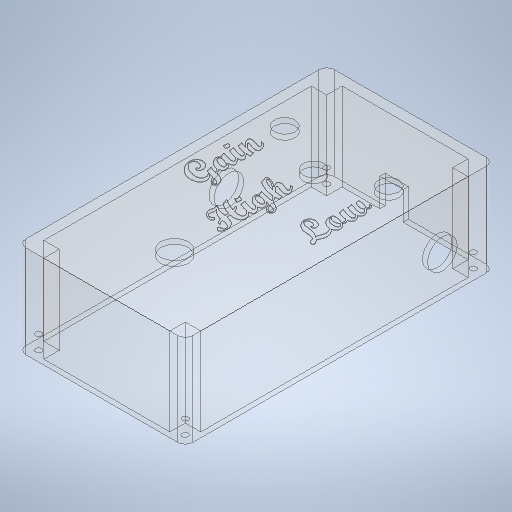
# Autodesk Inventor part: obudowa
Saved by Autodesk Inventor 2025 (Build 290162000, 162)
## iProperties
Created: 2026-04-02
Part Number: obudowa
Material: Tworzywo sztuczne PET
Document SubType Name: Modeling
Designer: zzapa
Density: 1.541 g/cm^3
Appearance: Poliwęglan — przezroczysty
Author: zzapa
Autodesk Inventor part; units mm, degrees
note: some values were not read from the file. Chosen so that the rebuilt part matches the saved one: direction of "JACK 2"; direction of "JACK 1".
ref_plane "YZ Plane" through (0, 0, 0) normal (1, 0, 0) x (0, 1, 0)
ref_plane "XZ Plane" through (0, 0, 0) normal (0, 1, 0) x (-1, 0, 0)
sketch "Szkic1" plane through (0, 0, 0) normal (0, 1, 0) x (-1, 0, 0)
  line L0 (65, -120) -> (0, -120)
  line L1 (0, -120) -> (0, 0)
  line L2 (0, 0) -> (65, 0)
  line L3 (65, 0) -> (65, -120)
  dimension "d0" = 120
  dimension "d1" = 65
  constraints: 8 end point, 2 parallel, 1 coincident, 1 horizontal, 1 perpendicular
  measures "d0" distance of L2.end L0.start
  measures "d1" distance of L0.start L0.end
extrude "Gabaryt" add sketch "Szkic1" along normal blind 36
ref_plane "Konstrukcja wycięcia" through (0, 34, 0) normal (0, 1, 0) x (1, 0, 0)
sketch "Szkic2" plane through (0, 0, 0) normal (0, -1, 0) x (1, 0, 0)
  line L0 (-65, 0) -> (0, 0) projected
  line L1 (-65, -120) -> (-65, 0) projected
  line L2 (0, -120) -> (-65, -120) projected
  line L3 (0, 0) -> (0, -120) projected
  line L4 (-2, -118) -> (-63, -118)
  line L5 (-63, -118) -> (-63, -2)
  line L6 (-63, -2) -> (-2, -2)
  line L7 (-2, -2) -> (-2, -118)
  dimension "d4" = 2
  constraints: 8 end point, 3 other
  measures "d4" distance between parallel lines of L3 L7
extrude "Wydrążenie" cut sketch "Szkic2" against normal up to surface (34 mm away) contours L4 L5 L6 L7
sketch "Szkic6" plane through (0, 0, 0) normal (0, -1, 0) x (1, 0, 0)
  line L0 (-65, 0) -> (0, 0) projected
  line L1 (-8, -8) -> (0, -8)
  line L2 (0, -8) -> (0, 0)
  line L3 (0, 0) -> (-8, 0)
  line L4 (-8, 0) -> (-8, -8)
  line L5 (0, 0) -> (0, -120) projected
  line L6 (0, -120) -> (-65, -120) projected
  line L7 (-65, -120) -> (-65, 0) projected
  line L8 (0, 0) -> (0, -120) projected
  line L9 (0, -60) -> (-65, -60)
  line L10 (-32.5, 0) -> (-32.5, -120)
  line L11 (-57, -8) -> (-65, -8)
  line L12 (-65, -8) -> (-65, 0)
  line L13 (-65, 0) -> (-57, 0)
  line L14 (-57, 0) -> (-57, -8)
  line L15 (-8, -112) -> (0, -112)
  line L16 (0, -112) -> (0, -120)
  line L17 (0, -120) -> (-8, -120)
  line L18 (-8, -120) -> (-8, -112)
  line L19 (-57, -112) -> (-65, -112)
  line L20 (-65, -112) -> (-65, -120)
  line L21 (-65, -120) -> (-57, -120)
  line L22 (-57, -120) -> (-57, -112)
  point P0 (-57, -120)
  point P1 (-65, -112)
  point P2 (-57, 0)
  point P3 (-8, -120)
  point P4 (0, -112)
  point P5 (-8, 0)
  dimension "d16" = 8
  dimension "d17" = 8
  constraints: 36 end point, 9 symmetric about line, 4 midpoint, 2 parallel, 1 horizontal, 1 perpendicular
  measures "d16" distance of L1.start L1.end
  measures "d17" distance of L3.end L1.start
extrude "Materiał na insert" add sketch "Szkic6" against normal up to surface (34 mm away) contours L0 L14 L11 L7 | L0 L2 L1 L4 | L19 L22 L6 L7 | L5 L6 L18 L15
sketch "Szkic7" plane through (0, 0, 0) normal (0, -1, 0) x (1, 0, 0)
  line L0 (0, 0) -> (0, -120) projected
  line L1 (0, -60) -> (-65, -60)
  line L2 (-65, -120) -> (-65, 0) projected
  line L3 (0, -120) -> (-65, -120) projected
  line L4 (-32.5, -120) -> (-32.5, 0)
  line L5 (-65, 0) -> (0, 0) projected
  point P0 (-4, -4)
  point P1 (-61, -4)
  point P2 (-4, -116)
  point P3 (-61, -116)
  dimension "d20" = 4
  dimension "d21" = 4
  constraints: 4 end point, 4 midpoint, 3 symmetric about line
  measures "d20" horizontal distance of L0.start point (-4, -4)
  measures "d21" horizontal distance of point (-4, -4) L0.start
hole "Otwory montażowe" at (-4, 0, -4) at (-61, 0, -4) at (-4, 0, -116) at (-61, 0, -116) direction (0, 1, 0) diameter 2.4 depth 5.5
fillet "Zaokrąglenie1" radius 3 4 edges at (-65, 18, 0) (0, 18, 0) (0, 18, -120) (-65, 18, -120)
sketch "Szkic8" plane through (-65, 0, -117) normal (-1, 0, 0) x (0, 0, 1)
  line L0 (-3, 36) -> (-3, 0) projected
  line L1 (0, 0) -> (114, 0) projected
  line L2 (0, 0) -> (-3, 0) projected
  line L3 (117, 0) -> (117, 36) projected
  point P0 (37, 15)
  dimension "d30" = 15
  dimension "d39" = 80
  measures "d30" distance from line of L1 point (37, 15)
  measures "d39" distance from line of L3 point (37, 15)
hole "JACK 1" at (-65, 15, -80) direction (1, 0, 0) diameter 11.5 depth 2
sketch "Szkic9" plane through (0, 0, -3) normal (1, 0, 0) x (0, 0, -1)
  line L0 (0, 0) -> (114, 0) projected
  line L1 (-3, 36) -> (-3, 0) projected
  point P0 (97, 15)
  dimension "d40" = 15
  dimension "d41" = 100
  measures "d40" distance from line of L0 point (97, 15)
  measures "d41" distance from line of point (97, 15) L1
hole "JACK 2" at (0, 15, -100) direction (-1, 0, 0) diameter 11.5 end up to surface
sketch "Szkic11" plane through (0, 36, 0) normal (0, 1, 0) x (1, 0, 0)
  circle A0 centre (-52.7305, 91.416) radius 4
  circle A1 centre (-32.5, 82.3712) radius 4
  line L0 (-3, 120) -> (-62, 120) projected
  line L1 (-32.5, 120) -> (-32.5, 0)
  line L2 (-62, 0) -> (-3, 0) projected
  circle A2 centre (-12.2695, 91.416) radius 4
  circle A3 centre (-32.5, 28.3603) radius 5.3281
  point P0 (0, 0)
  dimension "d51" = 8
  constraints: 4 centre point, 2 end point, 2 midpoint, 2 point on line, 1 equal radius, 1 symmetric about line, 1 other
  measures "d51" diameter of A0
extrude "Wyciągnięcie proste7" cut sketch "Szkic11" against normal up to surface (2 mm away)
sketch "Szkic12" plane through (-3, 0, -120) normal (0, 0, -1) x (-1, 0, 0)
  line L0 (0, 0) -> (59, 0) projected
  line L1 (30.3172, 11) -> (39.3172, 11)
  line L2 (39.3172, 11) -> (39.3172, 0)
  line L3 (39.3172, 0) -> (30.3172, 0)
  line L4 (30.3172, 0) -> (30.3172, 11)
  point P0 (-3, 0)
  point P1 (30.3172, 0)
  dimension "d54" = 11
  dimension "d55" = 9
  constraints: 8 end point, 2 parallel, 1 horizontal, 1 perpendicular, 1 point on line
  measures "d54" distance of L3.end L1.start
  measures "d55" distance of L1.start L1.end
extrude "Wyciągnięcie proste8" cut sketch "Szkic12" against normal up to surface (2 mm away)
sketch "Szkic13" plane through (0, 36, 0) normal (0, 1, 0) x (1, 0, 0)
  line L0 (-60.0879, 47.3044) -> (-60.0879, 81.416) construction
  line L1 (-60.0879, 81.416) -> (-45.3731, 81.416) construction
  line L2 (-45.3731, 81.416) -> (-45.3731, 47.3044) construction
  line L3 (-45.3731, 47.3044) -> (-60.0879, 47.3044) construction
  line L4 (-41.629, 38.2595) -> (-41.629, 72.3712) construction
  line L5 (-41.629, 72.3712) -> (-23.371, 72.3712) construction
  line L6 (-23.371, 72.3712) -> (-23.371, 38.2595) construction
  line L7 (-23.371, 38.2595) -> (-41.629, 38.2595) construction
  line L8 (-20.0288, 47.3044) -> (-20.0288, 81.416) construction
  line L9 (-20.0288, 81.416) -> (-4.5102, 81.416) construction
  line L10 (-4.5102, 81.416) -> (-4.5102, 47.3044) construction
  line L11 (-4.5102, 47.3044) -> (-20.0288, 47.3044) construction
  circle A0 centre (-52.7305, 91.416) radius 4 projected
  circle A1 centre (-32.5, 82.3712) radius 4 projected
  circle A2 centre (-12.2695, 91.416) radius 4 projected
  line L12 (-52.7305, 91.416) -> (-52.7305, 81.416)
  line L13 (-32.5, 82.3712) -> (-32.5, 72.3712)
  line L14 (-12.2695, 91.416) -> (-12.2695, 81.416)
  spline S0 degree 2 poles (-51.1094, 64.0031) (-50.5705, 63.5388) (-49.8905, 62.2121) knots 0 0 0 1 1 1
  spline S1 degree 2 poles (-49.8905, 62.2121) (-48.058, 61.9384) (-46.0514, 60.0479) (-46.0514, 58.8704) knots 0 0 0 1 2 2 2
  spline S2 degree 2 poles (-46.0514, 58.8704) (-46.0514, 58.3066) (-46.5738, 57.6681) (-47.0381, 57.6681) knots 0 0 0 1 2 2 2
  spline S3 degree 2 poles (-47.0381, 57.6681) (-48.3234, 57.6681) (-49.5257, 60.164) knots 0 0 0 1 1 1
  spline S4 degree 2 poles (-49.5257, 60.164) (-50.4544, 60.421) (-51.1924, 60.6698) knots 0 0 0 1 1 1
  spline S5 degree 2 poles (-51.1924, 60.6698) (-50.5705, 60.2303) (-49.6086, 58.5802) (-49.6086, 57.8671) knots 0 0 0 1 2 2 2
  spline S6 degree 2 poles (-49.6086, 57.8671) (-49.6086, 56.7063) (-51.6152, 55.1723) (-53.1492, 55.1723) knots 0 0 0 1 2 2 2
  spline S7 degree 2 poles (-53.1492, 55.1723) (-54.7661, 55.1723) (-57.6683, 56.9053) (-59.4096, 59.7328) (-59.4096, 61.0512) knots 0 0 0 1 2 3 3 3
  spline S8 degree 2 poles (-59.4096, 61.0512) (-59.4096, 62.2369) (-58.058, 63.7212) (-56.9801, 63.7212) knots 0 0 0 1 2 2 2
  spline S9 degree 2 poles (-56.9801, 63.7212) (-55.8275, 63.7212) (-54.0613, 62.0545) (-54.0613, 60.9766) knots 0 0 0 1 2 2 2
  spline S10 degree 2 poles (-54.0613, 60.9766) (-54.0613, 60.3381) (-54.6832, 59.5089) (-55.131, 59.5089) knots 0 0 0 1 2 2 2
  spline S11 degree 2 poles (-55.131, 59.5089) (-55.4129, 59.5089) (-55.8358, 59.8323) (-55.8358, 60.0479) knots 0 0 0 1 2 2 2
  spline S12 degree 2 poles (-55.8358, 60.0479) (-55.8358, 60.2552) (-55.5953, 60.2552) knots 0 0 0 1 1 1
  spline S13 degree 2 poles (-55.5953, 60.2552) (-55.3797, 60.2552) (-55.1476, 60.5703) (-55.1476, 60.7776) knots 0 0 0 1 2 2 2
  spline S14 degree 2 poles (-55.1476, 60.7776) (-55.1476, 61.3248) (-56.6567, 62.3364) (-57.5191, 62.3364) knots 0 0 0 1 2 2 2
  spline S15 degree 2 poles (-57.5191, 62.3364) (-58.1326, 62.3364) (-58.8955, 61.5487) (-58.8955, 60.9351) knots 0 0 0 1 2 2 2
  spline S16 degree 2 poles (-58.8955, 60.9351) (-58.8955, 59.9981) (-57.2454, 58.2568) (-54.5506, 57.1623) (-53.3317, 57.1623) knots 0 0 0 1 2 3 3 3
  spline S17 degree 2 poles (-53.3317, 57.1623) (-52.2205, 57.1623) (-50.9021, 58.1242) (-50.9021, 58.9202) knots 0 0 0 1 2 2 2
  spline S18 degree 2 poles (-50.9021, 58.9202) (-50.9021, 60.2718) (-52.8093, 61.5073) knots 0 0 0 1 1 1
  line L15 (-52.8093, 61.5073) -> (-52.9917, 62.8008)
  spline S19 degree 2 poles (-52.9917, 62.8008) (-53.0249, 63.0412) (-52.8756, 63.0412) knots 0 0 0 1 1 1
  spline S20 degree 2 poles (-52.8756, 63.0412) (-52.8093, 63.0412) (-51.7645, 62.6764) (-50.5373, 62.353) knots 0 0 0 1 2 2 2
  spline S21 degree 2 poles (-50.5373, 62.353) (-51.1509, 63.4227) (-51.9055, 64.0031) knots 0 0 0 1 1 1
  line L16 (-51.9055, 64.0031) -> (-51.1094, 64.0031)
  spline S22 degree 2 poles (-48.8292, 59.9981) (-47.9336, 58.2071) (-47.063, 58.2071) knots 0 0 0 1 1 1
  spline S23 degree 2 poles (-47.063, 58.2071) (-46.5987, 58.2071) (-46.5987, 58.6466) knots 0 0 0 1 1 1
  spline S24 degree 2 poles (-46.5987, 58.6466) (-46.5987, 59.5172) (-48.8292, 59.9981) knots 0 0 0 1 1 1
  spline S25 degree 2 poles (-51.1094, 71.3497) (-50.0647, 70.2469) (-49.4345, 69.2933) (-49.4345, 68.8621) knots 0 0 0 1 2 2 2
  spline S26 degree 2 poles (-49.4345, 68.8621) (-49.4345, 67.7759) (-51.3582, 67.834) knots 0 0 0 1 1 1
  spline S27 degree 2 poles (-51.3582, 67.834) (-50.3715, 67.1457) (-49.4345, 65.9849) (-49.4345, 65.363) knots 0 0 0 1 2 2 2
  spline S28 degree 2 poles (-49.4345, 65.363) (-49.4345, 64.7577) (-50.5705, 63.9119) (-51.3996, 63.9119) knots 0 0 0 1 2 2 2
  spline S29 degree 2 poles (-51.3996, 63.9119) (-52.4278, 63.9119) (-54.3018, 65.0479) (-55.4627, 66.8223) (-55.4627, 67.5023) knots 0 0 0 1 2 3 3 3
  spline S30 degree 2 poles (-55.4627, 67.5023) (-55.4627, 68.3646) (-54.6666, 68.7046) knots 0 0 0 1 1 1
  line L17 (-54.6666, 68.7046) -> (-55.4461, 70.1225)
  line L18 (-55.4461, 70.1225) -> (-55.4461, 70.5122)
  line L19 (-55.4461, 70.5122) -> (-53.4312, 69.8986)
  spline S31 degree 2 poles (-53.4312, 69.8986) (-51.9055, 69.426) (-51.3416, 69.426) knots 0 0 0 1 1 1
  spline S32 degree 2 poles (-51.3416, 69.426) (-50.7529, 69.426) (-50.7529, 69.8489) knots 0 0 0 1 1 1
  spline S33 degree 2 poles (-50.7529, 69.8489) (-50.7529, 70.1142) (-51.325, 70.761) (-51.9055, 71.3497) knots 0 0 0 1 2 2 2
  line L20 (-51.9055, 71.3497) -> (-51.1094, 71.3497)
  spline S34 degree 2 poles (-50.7363, 66.3082) (-50.7363, 66.9965) (-53.0829, 68.2154) (-54.0779, 68.2154) knots 0 0 0 1 2 2 2
  spline S35 degree 2 poles (-54.0779, 68.2154) (-54.4676, 68.2154) (-54.8988, 67.8671) (-54.8988, 67.5769) knots 0 0 0 1 2 2 2
  spline S36 degree 2 poles (-54.8988, 67.5769) (-54.8988, 66.8887) (-52.5522, 65.6615) (-51.5738, 65.6615) knots 0 0 0 1 2 2 2
  spline S37 degree 2 poles (-51.5738, 65.6615) (-51.2006, 65.6615) (-50.7363, 66.0263) (-50.7363, 66.3082) knots 0 0 0 1 2 2 2
  spline S38 degree 2 poles (-51.1094, 74.7328) (-49.4179, 73.1242) (-49.4179, 72.3199) knots 0 0 0 1 1 1
  spline S39 degree 2 poles (-49.4179, 72.3199) (-49.4179, 71.8804) (-50.3217, 71.2751) (-51.0016, 71.2751) knots 0 0 0 1 2 2 2
  spline S40 degree 2 poles (-51.0016, 71.2751) (-52.4693, 71.2751) (-55.0647, 72.2701) knots 0 0 0 1 1 1
  line L21 (-55.0647, 72.2701) -> (-55.4295, 74.0197)
  line L22 (-55.4295, 74.0197) -> (-55.4295, 74.1026)
  line L23 (-55.4295, 74.1026) -> (-53.2736, 73.4144)
  spline S41 degree 2 poles (-53.2736, 73.4144) (-51.9386, 72.9832) (-51.3665, 72.9832) knots 0 0 0 1 1 1
  spline S42 degree 2 poles (-51.3665, 72.9832) (-51.1426, 72.9832) (-50.8607, 73.1822) (-50.8607, 73.3315) knots 0 0 0 1 2 2 2
  spline S43 degree 2 poles (-50.8607, 73.3315) (-50.8607, 73.6051) (-51.2504, 74.1441) (-51.9055, 74.7328) knots 0 0 0 1 2 2 2
  line L24 (-51.9055, 74.7328) -> (-51.1094, 74.7328)
  spline S44 degree 2 poles (-58.1161, 74.5918) (-56.466, 74.5918) (-56.466, 73.3729) knots 0 0 0 1 1 1
  spline S45 degree 2 poles (-56.466, 73.3729) (-56.466, 72.7842) (-56.8225, 72.3613) knots 0 0 0 1 1 1
  spline S46 degree 2 poles (-56.8225, 72.3613) (-57.4278, 72.7593) (-58.1824, 72.9832) knots 0 0 0 1 1 1
  spline S47 degree 2 poles (-58.1824, 72.9832) (-57.8507, 73.5222) (-57.8507, 73.8539) knots 0 0 0 1 1 1
  spline S48 degree 2 poles (-57.8507, 73.8539) (-57.8507, 74.227) (-58.1161, 74.5918) knots 0 0 0 1 1 1
  spline S49 degree 2 poles (-51.1177, 81.499) (-49.4345, 79.9069) (-49.4345, 78.7709) knots 0 0 0 1 1 1
  spline S50 degree 2 poles (-49.4345, 78.7709) (-49.4345, 78.3066) (-50.0812, 77.7427) (-50.6285, 77.7427) knots 0 0 0 1 2 2 2
  spline S51 degree 2 poles (-50.6285, 77.7427) (-51.3665, 77.7427) (-52.8756, 78.348) knots 0 0 0 1 1 1
  spline S52 degree 2 poles (-52.8756, 78.348) (-53.6882, 78.6714) (-53.9038, 78.6714) knots 0 0 0 1 1 1
  spline S53 degree 2 poles (-53.9038, 78.6714) (-54.1277, 78.6714) (-54.1277, 78.4973) knots 0 0 0 1 1 1
  spline S54 degree 2 poles (-54.1277, 78.4973) (-54.1277, 78.4061) (-54.0282, 78.2485) knots 0 0 0 1 1 1
  spline S55 degree 2 poles (-54.0282, 78.2485) (-53.937, 78.0993) (-53.7628, 77.9086) knots 0 0 0 1 1 1
  spline S56 degree 2 poles (-53.7628, 77.9086) (-53.6053, 77.7345) (-53.3731, 77.5272) knots 0 0 0 1 1 1
  spline S57 degree 2 poles (-53.3731, 77.5272) (-53.1824, 77.3364) (-52.9336, 77.1291) knots 0 0 0 1 1 1
  line L25 (-52.9336, 77.1291) -> (-52.4859, 76.7394)
  spline S58 degree 2 poles (-52.4859, 76.7394) (-52.1791, 76.4907) (-51.8308, 76.4243) knots 0 0 0 1 1 1
  spline S59 degree 2 poles (-51.8308, 76.4243) (-51.2504, 76.3248) (-50.7612, 76.2834) knots 0 0 0 1 1 1
  spline S60 degree 2 poles (-50.7612, 76.2834) (-50.3963, 76.2668) (-49.7744, 76.2668) knots 0 0 0 1 1 1
  line L26 (-49.7744, 76.2668) -> (-49.4179, 74.7411)
  spline S61 degree 2 poles (-49.4179, 74.7411) (-50.3466, 74.6665) (-50.8026, 74.6665) knots 0 0 0 1 1 1
  spline S62 degree 2 poles (-50.8026, 74.6665) (-51.9137, 74.6665) (-53.8955, 75.1806) (-55.1393, 75.7527) knots 0 0 0 1 2 2 2
  line L27 (-55.1393, 75.7527) -> (-55.4627, 77.4359)
  spline S63 degree 2 poles (-55.4627, 77.4359) (-54.0365, 76.9053) (-53.2156, 76.7394) knots 0 0 0 1 1 1
  spline S64 degree 2 poles (-53.2156, 76.7394) (-54.4759, 77.8671) (-55.4461, 79.1938) (-55.4461, 79.7162) knots 0 0 0 1 2 2 2
  spline S65 degree 2 poles (-55.4461, 79.7162) (-55.4461, 80.0645) (-54.9154, 80.5288) (-54.5174, 80.5288) knots 0 0 0 1 2 2 2
  spline S66 degree 2 poles (-54.5174, 80.5288) (-53.854, 80.5288) (-52.3449, 79.9401) knots 0 0 0 1 1 1
  spline S67 degree 2 poles (-52.3449, 79.9401) (-51.3001, 79.5255) (-50.9933, 79.5255) knots 0 0 0 1 1 1
  spline S68 degree 2 poles (-50.9933, 79.5255) (-50.5788, 79.5255) (-50.5788, 79.8655) knots 0 0 0 1 1 1
  spline S69 degree 2 poles (-50.5788, 79.8655) (-50.5788, 80.3713) (-51.9055, 81.499) knots 0 0 0 1 1 1
  line L28 (-51.9055, 81.499) -> (-51.1177, 81.499)
  spline S70 degree 2 poles (-30.8541, 55.5553) (-29.9834, 54.7178) (-29.1708, 53.3413) (-29.1708, 52.6199) knots 0 0 0 1 2 2 2
  spline S71 degree 2 poles (-29.1708, 52.6199) (-29.1708, 51.8073) (-30.6053, 50.6962) (-31.9818, 50.6962) knots 0 0 0 1 2 2 2
  spline S72 degree 2 poles (-31.9818, 50.6962) (-32.5539, 50.6962) (-33.4826, 50.8455) knots 0 0 0 1 1 1
  spline S73 degree 2 poles (-33.4826, 50.8455) (-33.3997, 49.809) (-33.3831, 49.5768) knots 0 0 0 1 1 1
  spline S74 degree 2 poles (-33.3831, 49.5768) (-31.1111, 49.1374) (-29.1708, 46.9566) (-29.1708, 45.5719) knots 0 0 0 1 2 2 2
  spline S75 degree 2 poles (-29.1708, 45.5719) (-29.1708, 44.552) (-30.1161, 43.2335) (-30.5556, 43.2335) knots 0 0 0 1 2 2 2
  spline S76 degree 2 poles (-30.5556, 43.2335) (-30.8789, 43.2335) (-31.7081, 44.2203) (-31.7081, 44.411) knots 0 0 0 1 2 2 2
  spline S77 degree 2 poles (-31.7081, 44.411) (-31.7081, 44.6763) (-31.1277, 44.6763) knots 0 0 0 1 1 1
  spline S78 degree 2 poles (-31.1277, 44.6763) (-29.7098, 44.6763) (-29.7098, 45.6299) knots 0 0 0 1 1 1
  spline S79 degree 2 poles (-29.7098, 45.6299) (-29.7098, 46.3347) (-31.2769, 47.2634) (-33.1012, 47.5453) knots 0 0 0 1 2 2 2
  spline S80 degree 2 poles (-33.1012, 47.5453) (-32.9851, 46.7161) (-32.2968, 45.9035) knots 0 0 0 1 1 1
  spline S81 degree 2 poles (-32.2968, 45.9035) (-32.3715, 45.8455) (-32.8856, 45.804) knots 0 0 0 1 1 1
  spline S82 degree 2 poles (-32.8856, 45.804) (-33.6899, 46.5254) (-34.005, 47.7194) knots 0 0 0 1 1 1
  spline S83 degree 2 poles (-34.005, 47.7194) (-35.1161, 47.9599) (-36.5257, 48.6896) (-37.9934, 50.1821) knots 0 0 0 1 2 2 2
  spline S84 degree 2 poles (-37.9934, 50.1821) (-37.7114, 49.4607) (-37.7114, 49.0047) knots 0 0 0 1 1 1
  spline S85 degree 2 poles (-37.7114, 49.0047) (-37.7114, 48.7145) (-38.0265, 47.8272) (-38.0265, 47.5536) knots 0 0 0 1 2 2 2
  spline S86 degree 2 poles (-38.0265, 47.5536) (-38.0265, 46.9732) (-37.1808, 46.2269) (-36.7413, 46.2269) knots 0 0 0 1 2 2 2
  spline S87 degree 2 poles (-36.7413, 46.2269) (-36.3018, 46.2269) (-35.937, 46.6913) knots 0 0 0 1 1 1
  spline S88 degree 2 poles (-35.937, 46.6913) (-35.8043, 46.9068) (-35.6882, 46.9068) knots 0 0 0 1 1 1
  spline S89 degree 2 poles (-35.6882, 46.9068) (-35.4809, 46.9068) (-34.8673, 46.3513) (-34.8673, 46.1108) knots 0 0 0 1 2 2 2
  spline S90 degree 2 poles (-34.8673, 46.1108) (-34.8673, 45.8455) (-35.6302, 45.3894) (-36.0945, 45.3894) knots 0 0 0 1 2 2 2
  spline S91 degree 2 poles (-36.0945, 45.3894) (-37.1144, 45.3894) (-39.1625, 47.3878) (-39.1625, 48.3745) knots 0 0 0 1 2 2 2
  spline S92 degree 2 poles (-39.1625, 48.3745) (-39.1625, 48.5901) (-38.8143, 49.809) (-38.8143, 50.0329) knots 0 0 0 1 2 2 2
  spline S93 degree 2 poles (-38.8143, 50.0329) (-38.8143, 50.4723) (-39.1957, 50.8952) knots 0 0 0 1 1 1
  spline S94 degree 2 poles (-39.1957, 50.8952) (-38.9221, 51.4176) (-38.8474, 51.4176) knots 0 0 0 1 1 1
  spline S95 degree 2 poles (-38.8474, 51.4176) (-38.7562, 51.4176) (-37.9187, 50.5884) (-36.3765, 50.0578) (-34.2703, 49.7675) knots 0 0 0 1 2 3 3 3
  spline S96 degree 2 poles (-34.2703, 49.7675) (-34.3035, 50.5553) (-34.3947, 51.144) knots 0 0 0 1 1 1
  spline S97 degree 2 poles (-34.3947, 51.144) (-35.4643, 51.4508) (-36.9237, 52.1805) (-38.408, 53.1257) (-38.7313, 53.6316) (-39.1625, 55.2568) (-39.1625, 55.2651) knots 0 0 0 1 2 3 4 5 5 5
  spline S98 degree 2 poles (-39.1625, 55.2651) (-39.1625, 55.348) (-39.1211, 55.348) knots 0 0 0 1 1 1
  spline S99 degree 2 poles (-39.1211, 55.348) (-39.0216, 55.348) (-38.1592, 54.7261) (-35.9204, 53.5652) (-34.6517, 53.1755) knots 0 0 0 1 2 3 3 3
  spline S100 degree 2 poles (-34.6517, 53.1755) (-34.7678, 53.9218) (-35.3068, 54.6929) knots 0 0 0 1 1 1
  spline S101 degree 2 poles (-35.3068, 54.6929) (-35.2653, 54.7841) (-35.1078, 54.8256) (-34.7927, 54.8256) knots 0 0 0 1 2 2 2
  spline S102 degree 2 poles (-34.7927, 54.8256) (-34.0796, 54.2369) (-33.7811, 52.9267) knots 0 0 0 1 1 1
  spline S103 degree 2 poles (-33.7811, 52.9267) (-32.4295, 52.6365) (-31.874, 52.6365) knots 0 0 0 1 1 1
  spline S104 degree 2 poles (-31.874, 52.6365) (-31.194, 52.6365) (-30.4063, 53.2253) (-30.4063, 53.7228) knots 0 0 0 1 2 2 2
  spline S105 degree 2 poles (-30.4063, 53.7228) (-30.4063, 54.1208) (-30.9204, 54.9251) (-31.6501, 55.5553) knots 0 0 0 1 2 2 2
  line L29 (-31.6501, 55.5553) -> (-30.8541, 55.5553)
  spline S106 degree 2 poles (-30.8624, 58.9301) (-29.1708, 57.3214) (-29.1708, 56.5171) knots 0 0 0 1 1 1
  spline S107 degree 2 poles (-29.1708, 56.5171) (-29.1708, 56.0777) (-30.0746, 55.4723) (-30.7546, 55.4723) knots 0 0 0 1 2 2 2
  spline S108 degree 2 poles (-30.7546, 55.4723) (-32.2222, 55.4723) (-34.8176, 56.4674) knots 0 0 0 1 1 1
  line L30 (-34.8176, 56.4674) -> (-35.1824, 58.217)
  line L31 (-35.1824, 58.217) -> (-35.1824, 58.2999)
  line L32 (-35.1824, 58.2999) -> (-33.0265, 57.6117)
  spline S109 degree 2 poles (-33.0265, 57.6117) (-31.6915, 57.1805) (-31.1194, 57.1805) knots 0 0 0 1 1 1
  spline S110 degree 2 poles (-31.1194, 57.1805) (-30.8955, 57.1805) (-30.6136, 57.3795) (-30.6136, 57.5287) knots 0 0 0 1 2 2 2
  spline S111 degree 2 poles (-30.6136, 57.5287) (-30.6136, 57.8024) (-31.0033, 58.3413) (-31.6584, 58.9301) knots 0 0 0 1 2 2 2
  line L33 (-31.6584, 58.9301) -> (-30.8624, 58.9301)
  spline S112 degree 2 poles (-37.869, 58.7891) (-36.2189, 58.7891) (-36.2189, 57.5702) knots 0 0 0 1 1 1
  spline S113 degree 2 poles (-36.2189, 57.5702) (-36.2189, 56.9815) (-36.5755, 56.5586) knots 0 0 0 1 1 1
  spline S114 degree 2 poles (-36.5755, 56.5586) (-37.1808, 56.9566) (-37.9353, 57.1805) knots 0 0 0 1 1 1
  spline S115 degree 2 poles (-37.9353, 57.1805) (-37.6036, 57.7194) (-37.6036, 58.0511) knots 0 0 0 1 1 1
  spline S116 degree 2 poles (-37.6036, 58.0511) (-37.6036, 58.4243) (-37.869, 58.7891) knots 0 0 0 1 1 1
  spline S117 degree 2 poles (-30.8624, 65.6962) (-29.9502, 64.8173) (-29.5191, 63.5984) knots 0 0 0 1 1 1
  spline S118 degree 2 poles (-29.5191, 63.5984) (-27.7363, 63.0262) (-25.8043, 61.2684) (-25.8043, 60.2899) knots 0 0 0 1 2 2 2
  spline S119 degree 2 poles (-25.8043, 60.2899) (-25.8043, 59.751) (-26.476, 59.0876) (-27.0315, 59.0876) knots 0 0 0 1 2 2 2
  spline S120 degree 2 poles (-27.0315, 59.0876) (-27.7695, 59.0876) (-28.9386, 60.406) (-29.4859, 61.9815) knots 0 0 0 1 2 2 2
  line L34 (-29.4859, 61.9815) -> (-30.8458, 62.28)
  spline S121 degree 2 poles (-30.8458, 62.28) (-30.0995, 61.6166) (-29.403, 60.6548) (-29.403, 60.1655) knots 0 0 0 1 2 2 2
  spline S122 degree 2 poles (-29.403, 60.1655) (-29.403, 59.5934) (-30.4809, 58.8637) (-31.335, 58.8637) knots 0 0 0 1 2 2 2
  spline S123 degree 2 poles (-31.335, 58.8637) (-32.7446, 58.8637) (-35.199, 61.003) (-35.199, 62.2136) knots 0 0 0 1 2 2 2
  spline S124 degree 2 poles (-35.199, 62.2136) (-35.199, 62.877) (-34.6352, 63.3911) knots 0 0 0 1 1 1
  spline S125 degree 2 poles (-34.6352, 63.3911) (-34.743, 63.7062) (-34.9668, 64.2037) knots 0 0 0 1 1 1
  line L35 (-34.9668, 64.2037) -> (-35.1824, 64.6929)
  line L36 (-35.1824, 64.6929) -> (-35.1824, 64.8505)
  spline S126 degree 2 poles (-35.1824, 64.8505) (-34.3698, 64.5768) (-33.5987, 64.4359) knots 0 0 0 1 1 1
  line L37 (-33.5987, 64.4359) -> (-30.1493, 63.7891)
  spline S127 degree 2 poles (-30.1493, 63.7891) (-30.4975, 64.7178) (-31.6584, 65.6962) knots 0 0 0 1 1 1
  line L38 (-31.6584, 65.6962) -> (-30.8624, 65.6962)
  spline S128 degree 2 poles (-30.6468, 61.2601) (-30.6468, 61.7493) (-31.7993, 62.5039) (-33.5738, 62.9267) (-33.9221, 62.9267) knots 0 0 0 1 2 3 3 3
  spline S129 degree 2 poles (-33.9221, 62.9267) (-34.2371, 62.9267) (-34.66, 62.6034) (-34.66, 62.3629) knots 0 0 0 1 2 2 2
  spline S130 degree 2 poles (-34.66, 62.3629) (-34.66, 61.6332) (-32.6949, 60.547) (-31.675, 60.547) knots 0 0 0 1 2 2 2
  spline S131 degree 2 poles (-31.675, 60.547) (-31.2023, 60.547) (-30.6468, 60.9367) (-30.6468, 61.2601) knots 0 0 0 1 2 2 2
  spline S132 degree 2 poles (-28.8723, 61.8405) (-28.0763, 59.61) (-27.0315, 59.61) knots 0 0 0 1 1 1
  spline S133 degree 2 poles (-27.0315, 59.61) (-26.7164, 59.61) (-26.3267, 59.9831) (-26.3267, 60.2733) knots 0 0 0 1 2 2 2
  spline S134 degree 2 poles (-26.3267, 60.2733) (-26.3267, 60.7709) (-27.5788, 61.5005) (-28.8723, 61.8405) knots 0 0 0 1 2 2 2
  spline S135 degree 2 poles (-30.8624, 72.4541) (-29.1708, 70.8206) (-29.1708, 69.7675) knots 0 0 0 1 1 1
  spline S136 degree 2 poles (-29.1708, 69.7675) (-29.1708, 69.3032) (-29.8093, 68.6896) (-30.2985, 68.6896) knots 0 0 0 1 2 2 2
  spline S137 degree 2 poles (-30.2985, 68.6896) (-31.1277, 68.6896) (-32.6285, 69.3198) knots 0 0 0 1 1 1
  spline S138 degree 2 poles (-32.6285, 69.3198) (-33.4411, 69.6597) (-33.6899, 69.6597) knots 0 0 0 1 1 1
  spline S139 degree 2 poles (-33.6899, 69.6597) (-33.9718, 69.6597) (-33.9718, 69.3944) knots 0 0 0 1 1 1
  spline S140 degree 2 poles (-33.9718, 69.3944) (-33.9718, 69.1125) (-33.2255, 68.0677) (-32.5788, 67.4873) knots 0 0 0 1 2 2 2
  spline S141 degree 2 poles (-32.5788, 67.4873) (-31.3101, 67.2468) (-29.5274, 67.2468) knots 0 0 0 1 1 1
  line L39 (-29.5274, 67.2468) -> (-29.1708, 65.7128)
  spline S142 degree 2 poles (-29.1708, 65.7128) (-29.8922, 65.6216) (-30.738, 65.6216) knots 0 0 0 1 1 1
  spline S143 degree 2 poles (-30.738, 65.6216) (-32.7944, 65.6216) (-36.335, 66.7493) (-38.3167, 67.9599) knots 0 0 0 1 2 2 2
  spline S144 degree 2 poles (-38.3167, 67.9599) (-38.6816, 68.8637) (-39.1459, 70.207) (-39.1459, 70.2982) knots 0 0 0 1 2 2 2
  spline S145 degree 2 poles (-39.1459, 70.2982) (-39.1459, 70.4806) (-38.5655, 70.7294) (-38.1343, 70.7294) knots 0 0 0 1 2 2 2
  spline S146 degree 2 poles (-38.1343, 70.7294) (-37.4046, 70.7294) (-35.6302, 69.8339) (-34.3781, 68.8803) knots 0 0 0 1 2 2 2
  spline S147 degree 2 poles (-34.3781, 68.8803) (-34.9088, 69.8007) (-35.1824, 70.406) (-35.1824, 70.7294) knots 0 0 0 1 2 2 2
  spline S148 degree 2 poles (-35.1824, 70.7294) (-35.1824, 71.0777) (-34.6766, 71.5171) (-34.262, 71.5171) knots 0 0 0 1 2 2 2
  spline S149 degree 2 poles (-34.262, 71.5171) (-33.6401, 71.5171) (-31.0448, 70.5221) (-30.7131, 70.5221) knots 0 0 0 1 2 2 2
  spline S150 degree 2 poles (-30.7131, 70.5221) (-30.5638, 70.5221) (-30.3317, 70.7045) (-30.3317, 70.8289) knots 0 0 0 1 2 2 2
  spline S151 degree 2 poles (-30.3317, 70.8289) (-30.3317, 71.2684) (-31.6584, 72.4541) knots 0 0 0 1 1 1
  line L40 (-31.6584, 72.4541) -> (-30.8624, 72.4541)
  spline S152 degree 2 poles (-33.6899, 67.678) (-36.5506, 70.1407) (-37.9022, 70.1407) knots 0 0 0 1 1 1
  spline S153 degree 2 poles (-37.9022, 70.1407) (-38.3167, 70.1407) (-38.3167, 69.9168) knots 0 0 0 1 1 1
  spline S154 degree 2 poles (-38.3167, 69.9168) (-38.3167, 69.5354) (-35.6053, 68.1257) (-33.6899, 67.678) knots 0 0 0 1 2 2 2
  spline S155 degree 2 poles (-8.9652, 65.7776) (-7.3068, 64.1441) (-7.3068, 62.4359) knots 0 0 0 1 1 1
  spline S156 degree 2 poles (-7.3068, 62.4359) (-7.3068, 61.9384) (-7.5639, 61.0263) (-8.1609, 59.7079) (-8.3018, 59.2104) knots 0 0 0 1 2 3 3 3
  spline S157 degree 2 poles (-8.3018, 59.2104) (-7.2819, 58.2817) (-7.2819, 57.5272) knots 0 0 0 1 1 1
  spline S158 degree 2 poles (-7.2819, 57.5272) (-7.2819, 57.2701) (-7.6302, 56.9218) (-7.8707, 56.9218) knots 0 0 0 1 2 2 2
  spline S159 degree 2 poles (-7.8707, 56.9218) (-8.3931, 56.9218) (-9.1891, 57.95) (-9.3383, 58.887) knots 0 0 0 1 2 2 2
  spline S160 degree 2 poles (-9.3383, 58.887) (-9.8773, 59.2767) (-10.9055, 59.5006) (-12.0829, 59.5587) knots 0 0 0 1 2 2 2
  spline S161 degree 2 poles (-12.0829, 59.5587) (-14.5042, 59.6747) (-17.2571, 62.0379) (-17.2571, 63.4227) knots 0 0 0 1 2 2 2
  spline S162 degree 2 poles (-17.2571, 63.4227) (-17.2571, 64.3762) (-16.0547, 65.5951) (-15.1178, 65.5951) knots 0 0 0 1 2 2 2
  spline S163 degree 2 poles (-15.1178, 65.5951) (-14.0315, 65.5951) (-12.4063, 64.3182) (-12.4063, 63.4807) knots 0 0 0 1 2 2 2
  spline S164 degree 2 poles (-12.4063, 63.4807) (-12.4063, 63.0495) (-12.879, 62.552) (-13.2936, 62.552) knots 0 0 0 1 2 2 2
  spline S165 degree 2 poles (-13.2936, 62.552) (-13.5091, 62.552) (-13.7911, 62.6349) knots 0 0 0 1 1 1
  spline S166 degree 2 poles (-13.7911, 62.6349) (-13.5755, 62.8174) (-13.5755, 63.1076) knots 0 0 0 1 1 1
  spline S167 degree 2 poles (-13.5755, 63.1076) (-13.5755, 63.5719) (-14.6949, 64.2767) (-15.466, 64.2767) knots 0 0 0 1 2 2 2
  spline S168 degree 2 poles (-15.466, 64.2767) (-16.063, 64.2767) (-16.743, 63.7378) (-16.743, 63.2651) knots 0 0 0 1 2 2 2
  spline S169 degree 2 poles (-16.743, 63.2651) (-16.743, 62.7013) (-15.9304, 62.0711) (-14.7944, 61.8223) (-12.2737, 61.5487) (-10.3251, 60.8937) (-9.3881, 59.9898) knots 0 0 0 1 2 3 4 5 5 5
  spline S170 degree 2 poles (-9.3881, 59.9898) (-9.4295, 60.5786) (-9.214, 61.4409) (-8.6004, 63.0412) (-8.6004, 63.6217) knots 0 0 0 1 2 3 3 3
  spline S171 degree 2 poles (-8.6004, 63.6217) (-8.6004, 64.7494) (-9.7612, 65.7776) knots 0 0 0 1 1 1
  line L41 (-9.7612, 65.7776) -> (-8.9652, 65.7776)
  spline S172 degree 2 poles (-8.9569, 71.955) (-8.6501, 71.6068) (-8.4013, 70.9434) (-8.4013, 70.7527) knots 0 0 0 1 2 2 2
  spline S173 degree 2 poles (-8.4013, 70.7527) (-8.4013, 70.2552) (-8.7828, 69.766) knots 0 0 0 1 1 1
  spline S174 degree 2 poles (-8.7828, 69.766) (-7.2819, 68.7709) (-7.2819, 67.494) knots 0 0 0 1 1 1
  spline S175 degree 2 poles (-7.2819, 67.494) (-7.2819, 66.698) (-8.4843, 65.7029) (-9.471, 65.7029) knots 0 0 0 1 2 2 2
  spline S176 degree 2 poles (-9.471, 65.7029) (-11.0382, 65.7029) (-13.2936, 67.9335) (-13.2936, 69.484) knots 0 0 0 1 2 2 2
  spline S177 degree 2 poles (-13.2936, 69.484) (-13.2936, 70.0645) (-13.0365, 70.6117) (-12.6965, 70.7361) (-12.4312, 70.7361) knots 0 0 0 1 2 3 3 3
  spline S178 degree 2 poles (-12.4312, 70.7361) (-11.146, 70.7361) (-9.272, 70.0313) knots 0 0 0 1 1 1
  spline S179 degree 2 poles (-9.272, 70.0313) (-8.9486, 70.3879) (-8.9486, 70.7693) knots 0 0 0 1 1 1
  spline S180 degree 2 poles (-8.9486, 70.7693) (-8.9486, 71.2336) (-9.7529, 71.955) knots 0 0 0 1 1 1
  line L42 (-9.7529, 71.955) -> (-8.9569, 71.955)
  spline S181 degree 2 poles (-12.8126, 69.683) (-12.8541, 69.5752) (-12.8541, 69.3845) knots 0 0 0 1 1 1
  spline S182 degree 2 poles (-12.8541, 69.3845) (-12.8541, 68.489) (-10.9801, 67.4774) (-9.728, 67.4774) knots 0 0 0 1 2 2 2
  spline S183 degree 2 poles (-9.728, 67.4774) (-9.0315, 67.4774) (-8.2604, 67.9169) (-8.2604, 68.3149) knots 0 0 0 1 2 2 2
  spline S184 degree 2 poles (-8.2604, 68.3149) (-8.2604, 68.8041) (-9.1642, 69.3762) knots 0 0 0 1 1 1
  spline S185 degree 2 poles (-9.1642, 69.3762) (-9.9768, 68.7212) (-10.9138, 68.7212) knots 0 0 0 1 1 1
  spline S186 degree 2 poles (-10.9138, 68.7212) (-12.0166, 68.7212) (-12.8126, 69.683) knots 0 0 0 1 1 1
  spline S187 degree 2 poles (-8.9569, 81.499) (-8.6833, 81.1673) (-8.4511, 80.5039) (-8.4511, 80.3298) knots 0 0 0 1 2 2 2
  spline S188 degree 2 poles (-8.4511, 80.3298) (-8.4511, 79.824) (-8.8408, 79.3431) knots 0 0 0 1 1 1
  spline S189 degree 2 poles (-8.8408, 79.3431) (-7.2819, 78.091) (-7.2819, 76.7643) knots 0 0 0 1 1 1
  spline S190 degree 2 poles (-7.2819, 76.7643) (-7.2819, 75.7859) (-8.3599, 75.363) knots 0 0 0 1 1 1
  spline S191 degree 2 poles (-8.3599, 75.363) (-7.2819, 74.4426) (-7.2819, 73.3729) knots 0 0 0 1 1 1
  spline S192 degree 2 poles (-7.2819, 73.3729) (-7.2819, 72.6764) (-8.1941, 71.8804) (-9.0067, 71.8804) knots 0 0 0 1 2 2 2
  spline S193 degree 2 poles (-9.0067, 71.8804) (-9.869, 71.8804) (-11.6601, 72.3696) (-12.9536, 72.8754) knots 0 0 0 1 2 2 2
  line L43 (-12.9536, 72.8754) -> (-13.2936, 74.683)
  line L44 (-13.2936, 74.683) -> (-11.7596, 74.1772)
  spline S194 degree 2 poles (-11.7596, 74.1772) (-9.7612, 73.5305) (-8.9984, 73.5305) knots 0 0 0 1 1 1
  spline S195 degree 2 poles (-8.9984, 73.5305) (-8.6418, 73.5305) (-8.1858, 73.8787) (-8.1858, 74.1358) knots 0 0 0 1 2 2 2
  spline S196 degree 2 poles (-8.1858, 74.1358) (-8.1858, 74.6913) (-9.0481, 75.2386) knots 0 0 0 1 1 1
  spline S197 degree 2 poles (-9.0481, 75.2386) (-10.1261, 75.2386) (-11.2869, 75.6283) knots 0 0 0 1 1 1
  line L45 (-11.2869, 75.6283) -> (-12.9536, 76.1922)
  line L46 (-12.9536, 76.1922) -> (-13.2936, 78.0495)
  line L47 (-13.2936, 78.0495) -> (-10.9138, 77.2701)
  spline S198 degree 2 poles (-10.9138, 77.2701) (-9.7612, 76.897) (-9.0896, 76.897) knots 0 0 0 1 1 1
  spline S199 degree 2 poles (-9.0896, 76.897) (-8.6833, 76.897) (-8.2023, 77.2535) (-8.2023, 77.552) knots 0 0 0 1 2 2 2
  spline S200 degree 2 poles (-8.2023, 77.552) (-8.2023, 77.9169) (-8.7413, 78.5636) (-9.2886, 78.9699) knots 0 0 0 1 2 2 2
  spline S201 degree 2 poles (-9.2886, 78.9699) (-9.9519, 78.6051) (-10.6733, 78.6051) knots 0 0 0 1 1 1
  spline S202 degree 2 poles (-10.6733, 78.6051) (-11.7015, 78.6051) (-13.2936, 79.6416) (-13.2936, 80.2883) knots 0 0 0 1 2 2 2
  spline S203 degree 2 poles (-13.2936, 80.2883) (-13.2936, 80.7361) (-12.6219, 80.7361) knots 0 0 0 1 1 1
  spline S204 degree 2 poles (-12.6219, 80.7361) (-11.1625, 80.7361) (-9.33, 79.6084) knots 0 0 0 1 1 1
  spline S205 degree 2 poles (-9.33, 79.6084) (-8.9984, 79.9567) (-8.9984, 80.3381) knots 0 0 0 1 1 1
  spline S206 degree 2 poles (-8.9984, 80.3381) (-8.9984, 80.8024) (-9.7529, 81.499) knots 0 0 0 1 1 1
  line L48 (-9.7529, 81.499) -> (-8.9569, 81.499)
  point P0 (0, 0)
  dimension "d60" = 10
  constraints: 6 end point, 3 midpoint, 3 vertical, 2 parallel, 1 perpendicular, 6 other
  measures "d60" distance of L12.start L12.end
extrude "Napisy" cut sketch "Szkic13" against normal blind 0.2 contours L16 S21 S29 S30 L17 L18 L19 S31 S32 S33 L20 S40 S25 S26 S27 S28 S0 | S0 S28 S29 S21 L16 | S0 S1 S2 S3 S4 S5 S6 S7 S8 S9 S10 S11 S12 S13 S14 S15 S16 S17 S18 L15 S19 S20 S21 S29 S28 | S40 L20 S25 | S25 L20 S40 L21 L22 L23 S41 S42 S43 S62 S38 S39 | S62 L24 S38 | S38 L24 S62 L27 S63 S64 S65 S66 S67 S68 S69 L28 S49 S50 S51 S52 S53 S54 S55 S56 S57 L25 S58 S59 S60 L26 S61 | S44 S45 S46 S47 S48 | L29 S105 S108 L30 L31 L32 S109 S110 S111 S123 S122 S106 S107 S70 | S70 S108 S105 L29 | S70 S71 S72 S73 S74 S75 S76 S77 S78 S79 S80 S81 S82 S83 S84 S85 S86 S87 S88 S89 S90 S91 S92 S93 S94 S95 S96 S97 S98 S99 S100 S101 S102 S103 S104 S105 S108 | S122 S123 S111 L33 S106 | S106 L33 S111 S123 S124 S125 L35 L36 S126 L37 S127 S143 S117 S118 S119 S120 L34 S121 S122 | S143 S127 L38 S117 | S117 L38 S127 S143 S144 S145 S146 S147 S148 S149 S150 S151 L40 S135 S136 S137 S138 S139 S140 S141 L39 S142 | S112 S113 S114 S115 S116 | L41 S171 S176 S177 S178 S179 S180 S193 S192 S172 S173 S174 S175 S155 | S155 S175 S176 S171 L41 | S155 S156 S157 S158 S159 S160 S161 S162 S163 S164 S165 S166 S167 S168 S169 S170 S171 S176 S175 | S192 S193 S180 L42 S172 | S172 L42 S180 S193 L43 L44 S194 S195 S196 S197 L45 L46 L47 S198 S199 S200 S201 S202 S203 S204 S205 S206 L48 S187 S188 S189 S190 S191 S192
equation "\"d0\" = obudowa_a"
equation "\"d1\" = obudowa_b"
equation "\"d2\" = obudowa_wys"
equation "\"d4\" = obudowa_grubosc"
equation "\"d6\" = obudowa_wys"
equation "\"d16\" = obudowa_otwory_montazowe_material_x"
equation "\"d17\" = obudowa_otwory_montazowe_material_y"
equation "\"d20\" = obudowa_otwory_montazowe_poz_x"
equation "\"d21\" = obudowa_otwory_montazowe_poz_y"
equation "\"d22\" = insert_D"
equation "\"d24\" = gniazdo_M2_D1"
equation "\"d25\" = gniazdo_M2_glebokosc"
equation "\"d27\" = insert_glebokosc"
equation "\"d29\" = obudowa_zaokraglenie"
equation "\"d30\" = obudowa_otwory_io1_wys"
equation "\"d39\" = obudowa_otwory_io1_poz"
equation "\"d32\" = obudowa_otwory_io1_D"
equation "\"d37\" = insert_glebokosc"
equation "\"d40\" = obudowa_otwory_io2_wys"
equation "\"d41\" = obudowa_otwory_io2_poz"
equation "\"d42\" = obudowa_otwory_io2_D"
equation "\"d51\" = obudowa_otwory_pot_D"
equation "\"d54\" = input_wys"
equation "\"d55\" = input_a"
equation "\"gniazdo_M2_glebokosc\" = 1.5"
equation "\"gniazdo_M2_D1\" = 4.5"
equation "\"gniazdo_M2_D2\" = 2.6"
equation "\"podstawa_b\" = 65"
equation "\"podstawa_wys\" = 2"
equation "\"podstawa_otwory_montazowe_poz_x\" = 4"
equation "\"podstawa_otwory_montazowe_poz_y\" = 4"
equation "\"obudowa_b\" = 65"
equation "\"obudowa_a\" = 120"
equation "\"obudowa_wys\" = 36"
equation "\"obudowa_grubosc\" = 2"
equation "\"d5\" = -obudowa_grubosc"
equation "\"obudowa_prowadnica_odsuniecie\" = 2"
equation "\"obudowa_prowadnica_grubosc\" = 2"
equation "\"obudowa_kontrolki_a\" = 38"
equation "\"obudowa_prowadnica_wys\" = 19"
equation "\"obudowa_otwory_montazowe_poz_y\" = 4"
equation "\"obudowa_otwory_montazowe_poz_x\" = 4"
equation "\"obudowa_otwory_montazowe_material_y\" = 8"
equation "\"obudowa_otwory_montazowe_material_x\" = 8"
equation "\"insert_D\" = 2.4"
equation "\"insert_glebokosc\" = 5.5"
equation "\"obudowa_zaokraglenie\" = 3"
equation "\"podstawa_zaokraglenie\" = 3"
equation "\"obudowa_otwory_io_wys\" = 15"
equation "\"obudowa_otwory_io_D\" = 15"
equation "\"obudowa_otwory_io1_poz\" = 80"
equation "\"obudowa_otwory_io1_wys\" = 15"
equation "\"obudowa_otwory_io1_D\" = 11.5"
equation "\"obudowa_otwory_io2_poz\" = 100"
equation "\"obudowa_otwory_io2_wys\" = 15"
equation "\"obudowa_otwory_io2_D\" = 11.5"
equation "\"obudowa_otwory_pot_D\" = 8"
equation "\"input_b\" = 14.4"
equation "\"input_wys\" = 11"
equation "\"input_a\" = 9"
